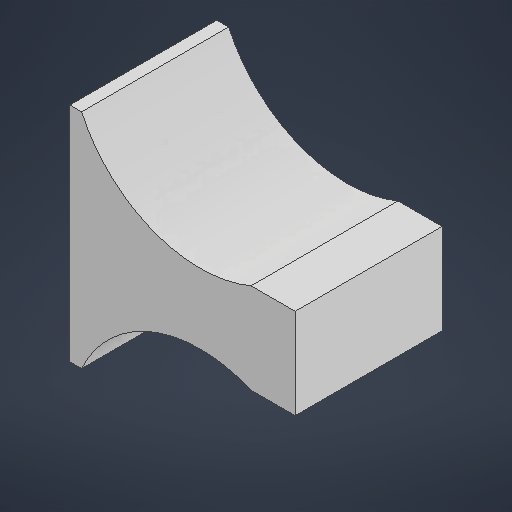
# Autodesk Inventor part: распорка
Saved by Autodesk Inventor 2025 (Build 290162000, 162)
## iProperties
Created: 2025-03-06
Part Number: распорка
Material: Типовые
Document SubType Name: Modeling
Designer: Phantom
Density: 1 g/cm^3
Appearance: По умолчанию
Author: Phantom
Autodesk Inventor part; units mm, degrees
ref_plane "YZ Plane" through (0, 0, 0) normal (1, 0, 0) x (0, 1, 0)
ref_plane "XZ Plane" through (0, 0, 0) normal (0, 1, 0) x (-1, 0, 0)
ref_plane "XY Plane" through (0, 0, 0) normal (0, 0, 1) x (1, 0, 0)
sketch "Эскиз1" plane through (0, 0, 0) normal (0, 0, 1) x (1, 0, 0)
  circle A0 centre (0, 0) radius 17.75
  line L0 (0, 0) -> (0, -45)
  circle A1 centre (0, -45) radius 17.75
  line L1 (12.9091, -12.1827) -> (12.9091, -32.8173)
  line L2 (-17.75, 0) -> (-17.75, -45)
  line L3 (9.8694, -14.7532) -> (14.166, -14.7532)
  line L4 (9.8694, -30.2468) -> (17.166, -30.2468)
  line L5 (-16.1446, -7.3766) -> (-17.75, -7.3766)
  line L6 (-16.1446, -37.6234) -> (-17.75, -37.6234)
  line L7 (6.9028, -16.3528) -> (15.2579, -16.3528)
  line L8 (6.9028, -28.6472) -> (17.9028, -28.6472)
  point P0 (12.9091, -30.2468)
  point P1 (12.9091, -14.7532)
  point P2 (12.9091, -28.6472)
  point P3 (12.9091, -16.3528)
  dimension "d0" = 35.5
  dimension "d1" = 45
  dimension "d2" = 35.5
  constraints: 18 end point, 10 point on circle, 3 horizontal, 3 perpendicular, 3 point on line, 2 centre point, 2 coincident, 2 vertical, 1 tangent
  measures "d0" diameter of A0
  measures "d1" distance of L0.start L0.end
  measures "d2" diameter of A1
extrude "Выдавливание1" add sketch "Эскиз1" along normal blind 20 contours A0 L0 A1 L6 L2 L5 | A0 L7 L1 L8 A1 L0
